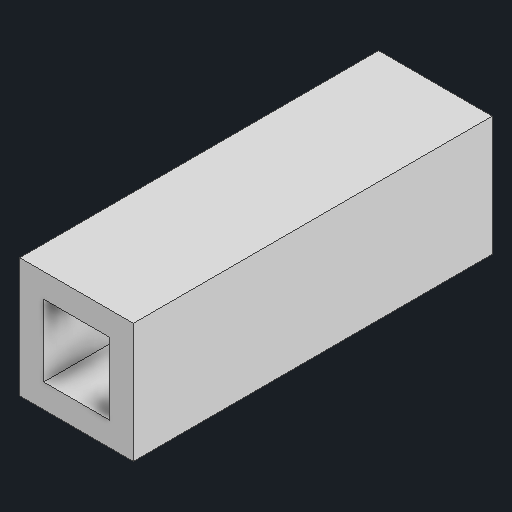
# Autodesk Inventor part: motorwheelstand
Saved by Autodesk Inventor 2026.2 (Build 302298000, 298)
## iProperties
Created: 2026-03-15
Part Number: motorwheelstand
Material: Generic
Document SubType Name: Modeling
Designer: danda
Density: 1 g/cm^3
Appearance: Default
Author: danda
Autodesk Inventor part; units mm, degrees
ref_plane "YZ Plane" through (0, 0, 0) normal (1, 0, 0) x (0, 1, 0)
ref_plane "XZ Plane" through (0, 0, 0) normal (0, 1, 0) x (-1, 0, 0)
ref_plane "XY Plane" through (0, 0, 0) normal (0, 0, 1) x (1, 0, 0)
sketch "Sketch1" plane through (0, 0, 0) normal (0, 0, 1) x (1, 0, 0)
  line L0 (27.3204, 31.1439) -> (38.3204, 31.1439)
  line L1 (38.3204, 31.1439) -> (38.3204, 19.1439)
  line L2 (38.3204, 19.1439) -> (27.3204, 19.1439)
  line L3 (27.3204, 19.1439) -> (27.3204, 31.1439)
  line L4 (42.3204, 35.1439) -> (23.3204, 35.1439)
  line L5 (23.3204, 35.1439) -> (23.3204, 15.1439)
  line L6 (23.3204, 15.1439) -> (42.3204, 15.1439)
  line L7 (42.3204, 15.1439) -> (42.3204, 35.1439)
  point P0 (0, 0)
  dimension "d0" = 11
  dimension "d1" = 12
  dimension "d2" = 4
  constraints: 16 end point, 4 parallel, 2 perpendicular, 1 horizontal, 3 other
  measures "d0" distance of L1.end L2.end
  measures "d1" distance of L0.end L1.end
  measures "d2" distance between parallel lines of L0 L4
extrude "Extrusion1" add sketch "Sketch1" along normal blind 60
body "Solid1"
